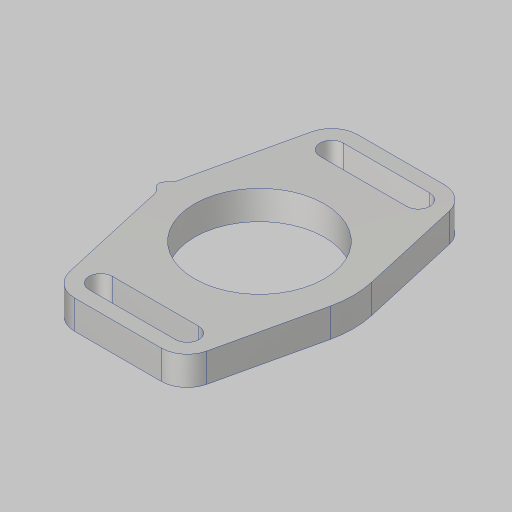
# Autodesk Inventor part: EL2-CGB-006
Saved by Autodesk Inventor 2023.5 (Build 275446000, 446)
## iProperties
Created: 2025-01-23
Part Number: EL2-CGB-006
Material: Aluminum 6061
Document SubType Name: Modeling
Designer: slick
Density: 2.7 g/cm^3
Appearance: Aluminum - Flat
Author: slick
Autodesk Inventor part; units mm, degrees
ref_plane "YZ Plane" through (0, 0, 0) normal (1, 0, 0) x (0, 1, 0)
ref_plane "XZ Plane" through (0, 0, 0) normal (0, 1, 0) x (-1, 0, 0)
ref_plane "XY Plane" through (0, 0, 0) normal (0, 0, 1) x (1, 0, 0)
sketch "Sketch1" plane through (0, 0, 0) normal (0, 1, 0) x (-1, 0, 0)
  circle A0 centre (0, 0) radius 14.2875
  line L0 (0, 25.4) -> (0, -25.4) construction
  circle A1 centre (0, 0) radius 18.1864 construction
  circle A2 centre (0, 25.4) radius 4.7625 construction
  circle A3 centre (0, -25.4) radius 4.7625 construction
  circle A4 centre (0, 0) radius 20.6375 construction
  line L1 (-9.525, -25.4) -> (9.525, -25.4) construction
  line L2 (-9.525, -27.9527) -> (9.525, -27.9527)
  line L3 (9.525, -22.8473) -> (-9.525, -22.8473)
  arc A5 (-9.525, -22.8473) -> (-9.525, -27.9527) centre (-9.525, -25.4) ccw
  arc A6 (9.525, -27.9527) -> (9.525, -22.8473) centre (9.525, -25.4) ccw
  line L4 (-9.525, 25.4) -> (9.525, 25.4) construction
  line L5 (-9.525, 22.8473) -> (9.525, 22.8473)
  line L6 (9.525, 27.9527) -> (-9.525, 27.9527)
  arc A7 (-9.525, 27.9527) -> (-9.525, 22.8473) centre (-9.525, 25.4) ccw
  arc A8 (9.525, 22.8473) -> (9.525, 27.9527) centre (9.525, 25.4) ccw
  line L7 (-9.525, -31.1277) -> (9.525, -31.1277)
  arc A9 (9.525, -31.1277) -> (9.525, -19.6723) centre (9.525, -25.4) ccw construction
  line L8 (9.525, -19.6723) -> (-9.525, -19.6723) construction
  arc A10 (-9.525, -19.6723) -> (-9.525, -31.1277) centre (-9.525, -25.4) ccw construction
  line L9 (-9.525, 31.1277) -> (9.525, 31.1277)
  arc A11 (9.525, 19.6723) -> (9.525, 31.1277) centre (9.525, 25.4) ccw construction
  line L10 (9.525, 19.6723) -> (-9.525, 19.6723) construction
  arc A12 (-9.525, 31.1277) -> (-9.525, 19.6723) centre (-9.525, 25.4) ccw construction
  line L11 (-15.1107, -26.6675) -> (-20.1258, -4.567)
  line L12 (15.1107, 26.6675) -> (20.1258, 4.567)
  line L13 (20.1258, -4.567) -> (15.1107, -26.6675)
  arc A13 (-15.1107, -26.6675) -> (-9.525, -31.1277) centre (-9.525, -25.4) ccw
  arc A14 (15.1107, 26.6675) -> (9.525, 31.1277) centre (9.525, 25.4) ccw
  arc A15 (9.525, -31.1277) -> (15.1107, -26.6675) centre (9.525, -25.4) ccw
  arc A16 (-20.1258, 4.567) -> (-20.1258, -4.567) centre (0, 0) ccw
  arc A17 (20.1258, -4.567) -> (20.1258, 4.567) centre (0, 0) ccw
  line L14 (-20.1258, 4.567) -> (-15.1107, 26.6675)
  arc A18 (-9.525, 31.1277) -> (-15.1107, 26.6675) centre (-9.525, 25.4) ccw
  point P0 (0, 25.4)
  dimension "d0" = 28.575
  dimension "d1" = 50.8
  dimension "d2" = 36.3728
  dimension "d3" = 9.525
  dimension "d4" = 9.525
  dimension "d5" = 6.35
  dimension "d20" = 5.1054
  dimension "d21" = 5.1054
  dimension "d22" = 19.05
  dimension "d25" = 3.175
  dimension "d26" = 3.175
  constraints: 36 point on circle, 34 end point, 19 centre point, 15 tangent, 14 coincident, 6 parallel, 3 midpoint, 3 vertical alignment, 1 concentric, 1 horizontal, 1 vertical, 6 other
  measures "d0" diameter of A0
  measures "d1" distance of L0.start L0.end
  measures "d2" diameter of A1
  measures "d3" diameter of A2
  measures "d4" diameter of A3
  measures "d5" radial gap between concentric circles of A0 A4
  measures "d20" diameter of A6
  measures "d21" diameter of A8
  measures "d22" distance of L1.start L1.end
  measures "d25" distance between parallel lines of L7 L2
  measures "d26" distance between parallel lines of L9 L6
extrude "Extrusion1" add sketch "Sketch1" along normal blind 6.35
hole "Hole1" at (0, 0, 25.4) at (0, 0, -25.4) direction (0, 1, 0) diameter 5.1054 end through all clearance for "Flat Head Machine Screw (82)" size "#10" standard "Ansi Unified Screw Threads"
sketch "Sketch2" plane through (0, 6.35, 0) normal (0, 1, 0) x (1, 0, 0)
  circle A0 centre (-20.955, 0) radius 1.1938
  circle A1 centre (0, 0) radius 14.2875 construction
  line L0 (9.525, -22.8473) -> (-9.525, -22.8473) projected
  arc A2 (-9.525, -22.8473) -> (-9.525, -27.9527) centre (-9.525, -25.4) ccw projected
  line L1 (-9.525, -27.9527) -> (9.525, -27.9527) projected
  arc A3 (9.525, -27.9527) -> (9.525, -22.8473) centre (9.525, -25.4) ccw projected
  line L2 (9.525, 27.9527) -> (-9.525, 27.9527) projected
  arc A4 (-9.525, 27.9527) -> (-9.525, 22.8473) centre (-9.525, 25.4) ccw projected
  line L3 (-9.525, 22.8473) -> (9.525, 22.8473) projected
  arc A5 (9.525, 22.8473) -> (9.525, 27.9527) centre (9.525, 25.4) ccw projected
  arc A6 (15.1107, 26.6675) -> (9.525, 31.1277) centre (9.525, 25.4) ccw projected
  line L4 (15.1107, 26.6675) -> (20.1258, 4.567) projected
  arc A7 (20.1258, -4.567) -> (20.1258, 4.567) centre (0, 0) ccw projected
  line L5 (20.1258, -4.567) -> (15.1107, -26.6675) projected
  arc A8 (9.525, -31.1277) -> (15.1107, -26.6675) centre (9.525, -25.4) ccw projected
  line L6 (9.525, -31.1277) -> (-9.525, -31.1277) projected
  arc A9 (-15.1107, -26.6675) -> (-9.525, -31.1277) centre (-9.525, -25.4) ccw projected
  line L7 (-15.1107, -26.6675) -> (-20.1258, -4.567) projected
  arc A10 (-20.1258, 4.567) -> (-20.1258, -4.567) centre (0, 0) ccw projected
  line L8 (-20.1258, 4.567) -> (-15.1107, 26.6675) projected
  arc A11 (-9.525, 31.1277) -> (-15.1107, 26.6675) centre (-9.525, 25.4) ccw projected
  line L9 (-9.525, 31.1277) -> (9.525, 31.1277) projected
  dimension "d15" = 2.3876
  dimension "d16" = 20.955
  constraints: 1 centre point
  measures "d15" diameter of A0
  measures "d16" distance of point (0, 0) A0.centre
extrude "Extrusion2" add sketch "Sketch2" against normal up to surface (6.35 mm away) contours A0 A10 | A10 A0
fillet "Fillet1" radius 3.175 2 edges at (-20.6059, 3.175, -1.1416) (-20.6059, 3.175, 1.1416)
body "Solid1"
